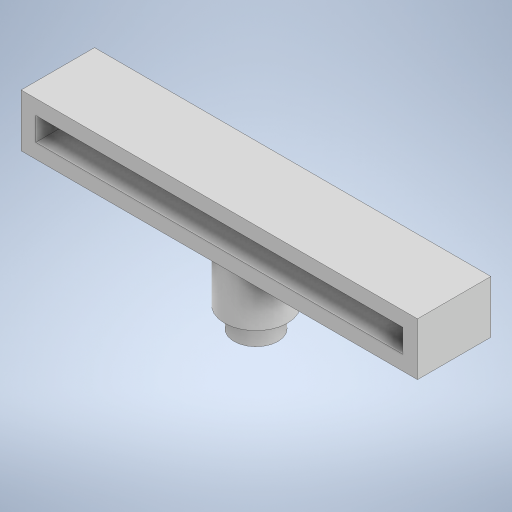
# Autodesk Inventor part: Bracket
Saved by Autodesk Inventor 2023 (Build 270158000, 158)
## iProperties
Created: 2023-03-23
Part Number: Bracket
Material: Generic
Document SubType Name: Modeling
Designer: bugme
Density: 1 g/cm^3
Appearance: Default
Author: bugme
Autodesk Inventor part; units mm, degrees
ref_plane "YZ Plane" through (0, 0, 0) normal (1, 0, 0) x (0, 1, 0)
ref_plane "XZ Plane" through (0, 0, 0) normal (0, 1, 0) x (-1, 0, 0)
ref_plane "XY Plane" through (0, 0, 0) normal (0, 0, 1) x (1, 0, 0)
sketch "Sketch1" plane through (0, 0, 0) normal (0, 0, 1) x (1, 0, 0)
  line L0 (-50, 20) -> (50, 20)
  line L1 (-50, 20) -> (-50, 13.65)
  line L2 (-50, 13.65) -> (50, 13.65)
  line L3 (50, 13.65) -> (50, 20)
  line L4 (54, 24) -> (-54, 24)
  line L5 (-54, 24) -> (-54, 9.65)
  line L6 (-54, 9.65) -> (54, 9.65)
  line L7 (54, 9.65) -> (54, 24)
  point P0 (0, 0)
  dimension "d0" = 100
  dimension "d1" = 6.35
  dimension "d2" = 4
  constraints: 16 end point, 4 perpendicular, 1 horizontal, 1 vertical, 3 other
  measures "d0" distance of L0.start L0.end
  measures "d1" distance of L0.start L1.end
  measures "d2" distance between parallel lines of L0 L4
extrude "Extrusion1" add sketch "Sketch1" along normal blind 20
sketch "Sketch2" plane through (-54, 9.65, 0) normal (0, -1, 0) x (1, 0, 0)
  circle A0 centre (54, 10) radius 6
  point P0 (54, 0)
  dimension "d5" = 12
  constraints: 1 centre point
  measures "d5" diameter of A0
extrude "Extrusion2" add sketch "Sketch2" along normal blind 20
sketch "Sketch3" plane through (-54, 9.65, 0) normal (0, -1, 0) x (1, 0, 0)
  circle A0 centre (54, 10) radius 6 projected
  circle A1 centre (54, 10) radius 8.5725
  point P0 (54, 0)
  dimension "d8" = 17.145
  constraints: 1 centre point, 1 coincident
  measures "d8" diameter of A1
extrude "Extrusion3" add sketch "Sketch3" along normal blind 14.4
body "Solid1"
